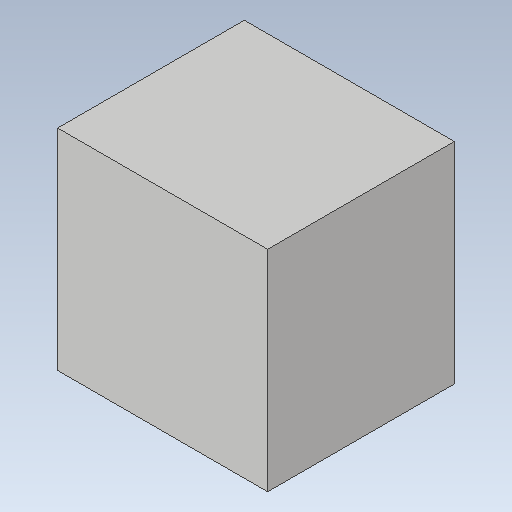
# Autodesk Inventor part: Gearbox
Saved by Autodesk Inventor 2020 (Build 240168000, 168)
## iProperties
Created: 2020-10-14
Part Number: Gearbox
Material: Generic
Document SubType Name: Modeling
Designer: nabee
Density: 1 g/cm^3
Appearance: Default
Author: nabee
Autodesk Inventor part; units mm, degrees
ref_plane "YZ Plane" through (0, 0, 0) normal (1, 0, 0) x (0, 1, 0)
ref_plane "XZ Plane" through (0, 0, 0) normal (0, 1, 0) x (-1, 0, 0)
ref_plane "XY Plane" through (0, 0, 0) normal (0, 0, 1) x (1, 0, 0)
sketch "Sketch1" plane through (0, 0, 0) normal (0, 0, 1) x (1, 0, 0)
  line L0 (0, 0) -> (180, 0)
  line L1 (180, 0) -> (180, 180)
  line L2 (180, 180) -> (0, 180)
  line L3 (0, 180) -> (0, 0)
  dimension "d0" = 180
  dimension "d1" = 180
  constraints: 8 end point, 2 parallel, 1 horizontal, 1 perpendicular
  measures "d0" distance of L0.start L0.end
  measures "d1" distance of L0.end L1.end
extrude "Extrusion1" add sketch "Sketch1" along normal blind 180
sketch "Sketch2" plane through (0, 0, 180) normal (0, 0, 1) x (1, 0, 0)
  line L0 (180, 180) -> (0, 180) projected
  line L1 (0, 0) -> (180, 0) projected
  line L2 (0, 180) -> (180, 180)
  line L3 (180, 180) -> (180, 0)
  line L4 (180, 0) -> (0, 0)
  line L5 (0, 0) -> (0, 180)
  constraints: 8 end point, 2 parallel, 1 horizontal, 1 perpendicular
extrude "Extrusion2" cut sketch "Sketch2" against normal blind 20
body "Solid1"
